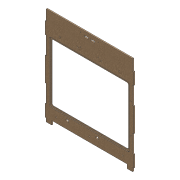
# Autodesk Inventor part: Frente Carcasa
Saved by Autodesk Inventor 2020 (Build 240168000, 168)
## iProperties
Created: 2020-06-04
Part Number: Frente Carcasa
Material: MDF Medium Density Fiberboard
Document SubType Name: Modeling
Designer: Dante
Density: 0.8 g/cm^3
Appearance: Cartón - Ondulado
Mass: 813.806 g
Surface Area: 2644.18 cm^2
Volume: 1017.26 cm^3
Author: Dante
Autodesk Inventor part; units mm, degrees
ref_plane "YZ Plane" through (0, 0, 0) normal (1, 0, 0) x (0, 1, 0)
ref_plane "XZ Plane" through (0, 0, 0) normal (0, 1, 0) x (-1, 0, 0)
ref_plane "XY Plane" through (0, 0, 0) normal (0, 0, 1) x (1, 0, 0)
sketch "Sketch1" plane through (0, 0, 0) normal (0, 0, 1) x (1, 0, 0)
  line L0 (72.9652, 2.3975) -> (452.9652, 2.3975)
  line L1 (479.9652, 474.8975) -> (45.9652, 474.8975)
  line L2 (479.9652, -17.6025) -> (452.9652, -17.6025)
  line L3 (452.9652, -17.6025) -> (452.9652, 2.3975)
  line L4 (45.9652, -17.6025) -> (72.9652, -17.6025)
  line L5 (72.9652, -17.6025) -> (72.9652, 2.3975)
  line L6 (479.9652, 474.8975) -> (479.9652, 474.9415)
  line L7 (45.9652, 474.8975) -> (45.9652, 474.8975)
  line L8 (479.9652, 59.8925) -> (479.9652, 59.8925)
  line L9 (455.9652, 57.3975) -> (69.9652, 57.3975)
  line L10 (45.9652, 474.8975) -> (45.9652, 474.8975)
  line L11 (36.9652, 522.3965) -> (36.9552, 522.3965)
  line L12 (463.9652, 65.3975) -> (463.9652, 355.3975)
  line L13 (61.9652, 65.3975) -> (61.9652, 355.3975)
  line L14 (455.9652, 347.3975) -> (455.9652, 73.3975)
  line L15 (447.9652, 65.3975) -> (77.9652, 65.3975)
  line L16 (69.9652, 73.3975) -> (69.9652, 347.3975)
  arc A0 (69.9652, 363.3975) -> (61.9652, 355.3975) centre (69.9652, 355.3975) ccw
  arc A1 (77.9652, 355.3975) -> (69.9652, 347.3975) centre (77.9652, 347.3975) ccw
  arc A2 (61.9652, 65.3975) -> (69.9652, 57.3975) centre (69.9652, 65.3975) ccw
  arc A3 (69.9652, 73.3975) -> (77.9652, 65.3975) centre (77.9652, 73.3975) ccw
  arc A4 (455.9652, 57.3975) -> (463.9652, 65.3975) centre (455.9652, 65.3975) ccw
  arc A5 (447.9652, 65.3975) -> (455.9652, 73.3975) centre (447.9652, 73.3975) ccw
  arc A6 (455.9652, 347.3975) -> (447.9652, 355.3975) centre (447.9652, 347.3975) ccw
  arc A7 (463.9652, 355.3975) -> (455.9652, 363.3975) centre (455.9652, 355.3975) ccw
  line L17 (69.9652, 363.3975) -> (455.9652, 363.3975)
  line L18 (447.9652, 355.3975) -> (77.9652, 355.3975)
  line L19 (479.9652, 150.3975) -> (485.4652, 150.3975)
  line L20 (479.9652, 270.3975) -> (485.4652, 270.3975)
  line L21 (485.4652, 270.3975) -> (485.4652, 150.3975)
  line L22 (40.4652, 270.3975) -> (40.4652, 150.3975)
  line L23 (40.4652, 150.3975) -> (45.9652, 150.3975)
  line L24 (40.4652, 270.3975) -> (45.9652, 270.3975)
  circle A8 centre (95.9652, 27.3975) radius 3
  circle A9 centre (429.9652, 27.3975) radius 3
  circle A10 centre (412.4652, 386.0395) radius 3
  circle A11 centre (113.4652, 386.0395) radius 3
  circle A12 centre (322.4652, 386.0395) radius 3
  circle A13 centre (203.4652, 386.0395) radius 3
  circle A14 centre (262.9652, 27.3975) radius 3
  circle A15 centre (471.4652, 135.3975) radius 2
  circle A16 centre (471.4652, 285.3975) radius 2
  line L25 (45.9652, 270.3975) -> (45.9652, 360.3975)
  line L26 (45.9652, 360.3975) -> (40.4652, 360.3975)
  line L27 (40.4652, 360.3975) -> (40.4652, 420.3975)
  line L28 (40.4652, 420.3975) -> (45.9652, 420.3975)
  line L29 (45.9652, 474.8975) -> (45.9652, 420.3975)
  line L30 (45.9652, 360.3975) -> (45.9652, 270.3975)
  line L31 (45.9652, 150.3975) -> (45.9652, 60.3975)
  line L32 (45.9652, 60.3975) -> (40.4652, 60.3975)
  line L33 (40.4652, 60.3975) -> (40.4652, 0.3975)
  line L34 (40.4652, 0.3975) -> (45.9652, 0.3975)
  line L35 (45.9652, 150.3975) -> (45.9652, 60.3975)
  line L36 (45.9652, 0.3975) -> (45.9652, -17.6025)
  line L37 (479.9652, 360.3975) -> (485.4652, 360.3975)
  line L38 (485.4652, 360.3975) -> (485.4652, 420.3975)
  line L39 (485.4652, 420.3975) -> (479.9652, 420.3975)
  line L40 (479.9652, 474.8975) -> (479.9652, 420.3975)
  line L41 (479.9652, 150.3975) -> (479.9652, 60.3975)
  line L42 (479.9652, 60.3975) -> (485.4652, 60.3975)
  line L43 (485.4652, 60.3975) -> (485.4652, 0.3975)
  line L44 (485.4652, 0.3975) -> (479.9652, 0.3975)
  line L45 (479.9652, -17.6025) -> (479.9652, 0.3975)
  line L46 (479.9652, 60.3975) -> (479.9652, 150.3975)
  line L47 (479.9652, 270.3975) -> (479.9652, 360.3975)
  line L48 (262.9652, 474.8975) -> (262.9652, 460.0682)
  circle A17 centre (218.9652, 459.8975) radius 1.5
  circle A18 centre (218.9652, 394.8975) radius 1.5
  circle A19 centre (306.9652, 459.8975) radius 1.5
  circle A20 centre (306.9652, 394.8975) radius 1.5
  line L49 (268.2652, 455.7975) -> (289.5652, 455.7975)
  line L50 (289.5652, 455.7975) -> (289.5652, 446.7975)
  line L51 (289.5652, 446.7975) -> (268.2652, 446.7975)
  line L52 (268.2652, 446.7975) -> (268.2652, 455.7975)
  line L53 (236.3652, 455.7975) -> (257.6652, 455.7975)
  line L54 (257.6652, 455.7975) -> (257.6652, 446.7975)
  line L55 (257.6652, 446.7975) -> (236.3652, 446.7975)
  line L56 (236.3652, 446.7975) -> (236.3652, 455.7975)
  point P0 (77.9853, 6.3978)
  point P1 (463.9652, 57.3975)
  dimension "d36" = 492.5
  dimension "d148" = 55
  dimension "d182" = 8
  dimension "d184" = 380
  dimension "d187" = 434
  dimension "d191" = 8
  dimension "d192" = 8
  dimension "d193" = 8
  dimension "d194" = 8
  dimension "d195" = 8
  dimension "d196" = 386
  dimension "d197" = 370
  dimension "d198" = 8
  dimension "d201" = 8
  dimension "d202" = 8
  dimension "d203" = 370
  dimension "d204" = 386
  dimension "d205" = 290
  dimension "d206" = 298
  dimension "d211" = 168
  dimension "d212" = 5.5
  dimension "d214" = 5.5
  dimension "d218" = 120
  dimension "d220" = 6
  dimension "d222" = 38
  dimension "d229" = 6
  dimension "d230" = 38
  dimension "d234" = 6
  dimension "d235" = 6
  dimension "d238" = 6
  dimension "d239" = 6
  dimension "d242" = 38
  dimension "d243" = 4
  dimension "d245" = 4
  dimension "d247" = 150
  dimension "d248" = 153
  dimension "d249" = 88.858
  dimension "d251" = 88.858
  dimension "d253" = 88.858
  dimension "d254" = 90
  dimension "d256" = 90
  dimension "d257" = 90
  dimension "d258" = 60
  dimension "d259" = 90
  dimension "d260" = 5.5
  dimension "d261" = 60
  dimension "d262" = 90
  dimension "d263" = 5.5
  dimension "d264" = 60
  dimension "d265" = 90
  dimension "d266" = 60
  dimension "d267" = 120
  dimension "d268" = 90
  dimension "d270" = 3
  dimension "d271" = 44
  dimension "d272" = 15
  dimension "d273" = 3
  dimension "d274" = 65
  dimension "d275" = 88
  dimension "d282" = 19.1
  dimension "d283" = 21.3
  dimension "d284" = 5.3
  dimension "d285" = 21.3
  dimension "d286" = 5.3
  constraints: 114 end point, 26 perpendicular, 21 centre point, 16 point on circle, 13 parallel, 11 tangent, 7 equal radius, 7 vertical, 6 horizontal, 3 point on line, 2 symmetric about line, 1 midpoint, 2 other
  measures "d36" distance between parallel lines of L2 L1
  measures "d148" distance between parallel lines of L0 L9
  measures "d182" radius of A0
  measures "d184" distance from line of L2.end L5
  measures "d187" distance of L2.start L4.start
  measures "d191" distance between parallel lines of L9 L15
  measures "d192" distance between parallel lines of L12 L14
  measures "d193" radius of A5
  measures "d194" radius of A4
  measures "d195" radius of A2
  measures "d196" distance of L9.start L9.end
  measures "d197" distance of L15.start L15.end
  measures "d198" distance between parallel lines of L13 L16
  measures "d201" radius of A3
  measures "d202" radius of A1
  measures "d203" distance of L18.start L18.end
  measures "d204" distance of L17.start L17.end
  measures "d205" distance between parallel lines of L18 L15
  measures "d206" distance between parallel lines of L17 L15
  measures "d211" distance of L2.start L19.start
  measures "d212" distance of L19.start L19.end
  measures "d214" distance of L20.start L20.end
  measures "d218" distance of L22.start L22.end
  measures "d220" diameter of A8
  measures "d222" distance from line of L15 A8.centre
  measures "d229" diameter of A9
  measures "d230" distance from line of L15 A9.centre
  measures "d234" diameter of A10
  measures "d235" diameter of A11
  measures "d238" diameter of A12
  measures "d239" diameter of A13
  measures "d242" distance from line of L15 A14.centre
  measures "d243" diameter of A15
  measures "d245" diameter of A16
  measures "d247" distance of A15.centre A16.centre
  measures "d248" distance from line of L2 A15.centre
  measures "d249" distance from line of L1 A11.centre
  measures "d251" distance from line of L1 A12.centre
  measures "d253" distance from line of L1 A10.centre
  measures "d254" distance of A10.centre A12.centre
  measures "d256" distance of A13.centre A11.centre
  measures "d257" distance of L24.end L25.end
  measures "d258" distance of L26.end L27.end
  measures "d259" distance of L23.end L31.end
  measures "d260" distance of L31.end L32.end
  measures "d261" distance of L32.end L33.end
  measures "d262" distance of L20.start L37.start
  measures "d263" distance of L37.start L37.end
  measures "d264" distance of L37.end L38.end
  measures "d265" distance of L19.start L41.end
  measures "d266" distance of L42.end L43.end
  measures "d267" distance of L20.end L19.end
  measures "d268" distance of L20.start L37.start
  measures "d270" diameter of A17
  measures "d271" distance from line of A17.centre L48
  measures "d272" distance from line of L1 A17.centre
  measures "d273" diameter of A18
  measures "d274" distance of A18.centre A17.centre
  measures "d275" distance of A18.centre A20.centre
  measures "d282" distance between parallel lines of L49 L1
  measures "d283" distance between parallel lines of L50 L52
  measures "d284" distance between parallel lines of L48 L52
  measures "d285" distance between parallel lines of L54 L56
  measures "d286" distance between parallel lines of L54 L48
extrude "Extrusion6" add sketch "Sketch1" along normal blind 5.5 contours L5 L4 L36 L34 L33 L32 L31 L23 L22 L24 L25 L26 L27 L28 L29 L1 L40 L39 L38 L37 L47 L20 L21 L19 L41 L42 L43 L44 L45 L2 L3 L0
extrude "Extrusión9" add sketch "Sketch1" along normal blind 2.5 contours L9 A2 L13 A0 L17 A7 L12 A4
sketch "Boceto2" plane through (0, 0, 5.5) normal (0, 0, 1) x (1, 0, 0)
  line L0 (72.9652, 2.3975) -> (452.9652, 2.3975) projected
  circle A0 centre (150.9652, 40.3975) radius 7
  circle A1 centre (300.9652, 40.3975) radius 7
  line L1 (45.9652, 150.3975) -> (45.9652, 60.3975) projected
  line L2 (45.9652, 60.3975) -> (45.9652, 2.3975)
  dimension "d159" = 14
  dimension "d162" = 14
  dimension "d165" = 150
  dimension "d269" = 105
  constraints: 2 centre point, 2 end point, 1 vertical
  measures "d159" diameter of A0
  measures "d162" diameter of A1
  measures "d165" distance of A1.centre A0.centre
  measures "d269" distance from line of L2 A0.centre
extrude "Extrusión10" cut sketch "Boceto2" against normal blind 9
body "Solid3"
